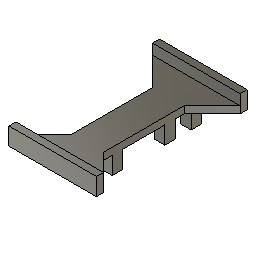
v2 (Autodesk Fusion 360 design; units mm, degrees)
Autodesk Fusion 360 part; units mm, degrees
sketch "Sketch1" plane through (0, 0, 0) normal (0, 0, 1) x (1, 0, 0) in component "Component'"
  line L0 (-12.5, 21.5) -> (12.5, 21.5)
  line L1 (12.5, 21.5) -> (12.5, 19.5)
  line L2 (12.5, 19.5) -> (-12.5, 19.5)
  line L3 (-12.5, 19.5) -> (-12.5, 21.5)
  line L4 (-12.5, -19.5) -> (12.5, -19.5)
  line L5 (12.5, -19.5) -> (12.5, -21.5)
  line L6 (12.5, -21.5) -> (-12.5, -21.5)
  line L7 (-12.5, -21.5) -> (-12.5, -19.5)
  line L8 (0, -19.5) -> (0, 19.5) construction
  line L9 (-4.5, 9) -> (-1.5, 9)
  line L10 (-1.5, 9) -> (-1.5, 6)
  line L11 (-1.5, 6) -> (-4.5, 6)
  line L12 (-4.5, 6) -> (-4.5, 9)
  line L13 (-1.5, 16.5) -> (-1.5, 13.5)
  line L14 (-1.5, 13.5) -> (-4.5, 13.5)
  line L15 (-4.5, 13.5) -> (-4.5, 16.5)
  line L16 (-4.5, 16.5) -> (-1.5, 16.5)
  line L17 (-4.5, -16.5) -> (-4.5, -13.5)
  line L18 (-1.5, -6) -> (-1.5, -9)
  line L19 (-4.5, -6) -> (-1.5, -6)
  line L20 (-4.5, -13.5) -> (-1.5, -13.5)
  line L21 (-4.5, -9) -> (-4.5, -6)
  line L22 (-1.5, -16.5) -> (-4.5, -16.5)
  line L23 (-1.5, -9) -> (-4.5, -9)
  line L24 (-1.5, -13.5) -> (-1.5, -16.5)
  line L25 (-20, 0) -> (15, 0) construction
  line L26 (4.5, 9) -> (4.5, 6)
  line L27 (4.5, 16.5) -> (4.5, 13.5)
  line L28 (1.5, 13.5) -> (1.5, 16.5)
  line L29 (4.5, -16.5) -> (1.5, -16.5)
  line L30 (4.5, -13.5) -> (4.5, -16.5)
  line L31 (1.5, -6) -> (4.5, -6)
  line L32 (4.5, -6) -> (4.5, -9)
  line L33 (1.5, -9) -> (1.5, -6)
  line L34 (1.5, -16.5) -> (1.5, -13.5)
  line L35 (1.5, 6) -> (1.5, 9)
  line L36 (1.5, 9) -> (4.5, 9)
  line L37 (4.5, 6) -> (1.5, 6)
  line L38 (4.5, -9) -> (1.5, -9)
  line L39 (1.5, 16.5) -> (4.5, 16.5)
  line L40 (1.5, -13.5) -> (4.5, -13.5)
  line L41 (4.5, 13.5) -> (1.5, 13.5)
  line L42 (4.5, 19.5) -> (4.5, -19.5)
  line L43 (-4.5, 19.5) -> (-4.5, -19.5)
  line L44 (12.5, 19.5) -> (4.5, 11.5)
  line L45 (12.5, 19.5) -> (24.453, 19.5) construction
  line L46 (-12.5, 19.5) -> (-4.5, 11.5)
  line L47 (-12.5, -19.5) -> (-4.5, -11.5)
  line L48 (12.5, -19.5) -> (4.5, -11.5)
  dimension "d1" = 39
  dimension "d2" = 25
  dimension "d3" = 2
  dimension "d6" = 3
  dimension "d7" = 3
  dimension "d8" = 1.5
  dimension "d9" = 7.5
  dimension "d10" = 3
  dimension "d11" = 3
  dimension "d12" = 7.5
  dimension "d13" = 12
  dimension "d14" = 3
  dimension "d15" = 3
  dimension "d16" = 7.5
  dimension "d17" = 3
  dimension "d18" = 3
  dimension "d19" = 7.5
  dimension "d20" = 12
  dimension "d21" = 135
  constraint horizontal L0
  constraint vertical L1
  constraint horizontal L2
  constraint vertical L3
  constraint horizontal L4
  constraint vertical L5
  constraint horizontal L6
  constraint vertical L7
  constraint equal L2 L4
  constraint equal L3 L7
  constraint coincident L4 L8.start
  constraint midpoint L2 L8.end
  constraint midpoint L4 L8.start
  constraint vertical L8
  constraint midpoint origin L8
  constraint horizontal L9
  constraint vertical L10
  constraint horizontal L11
  constraint vertical L12
  constraint horizontal L16
  constraint vertical L13
  constraint horizontal L14
  constraint vertical L15
  constraint equal L9 L16
  constraint equal L12 L15
  constraint horizontal L20
  constraint vertical L24
  constraint horizontal L22
  constraint vertical L17
  constraint horizontal L19
  constraint vertical L18
  constraint horizontal L23
  constraint vertical L21
  constraint equal L19 L20
  constraint equal L17 L21
  constraint horizontal L25
  constraint symmetric L11 L19 L25
  constraint collinear L10 L13
  constraint collinear L18 L24
  constraint collinear L10 L18
  constraint horizontal L36
  constraint vertical L26
  constraint horizontal L37
  constraint vertical L35
  constraint horizontal L39
  constraint vertical L27
  constraint horizontal L41
  constraint vertical L28
  constraint equal L36 L39
  constraint equal L28 L35
  constraint horizontal L40
  constraint vertical L30
  constraint horizontal L29
  constraint vertical L34
  constraint horizontal L31
  constraint vertical L32
  constraint horizontal L38
  constraint vertical L33
  constraint equal L31 L40
  constraint equal L33 L34
  constraint collinear L26 L27
  constraint collinear L30 L32
  constraint collinear L26 L32
  constraint symmetric L8 L10 L35
  constraint collinear L11 L37
  constraint coincident L2 L42.start
  constraint coincident L4 L42.end
  constraint perpendicular L4 L42
  constraint coincident L2 L43.start
  constraint coincident L4 L43.end
  constraint perpendicular L4 L43
  constraint collinear L26 L42
  constraint horizontal L45
  constraint coincident L42 L44.end
  constraint coincident L43 L46.end
  constraint coincident L43 L47.end
  constraint coincident L42 L48.end
  constraint symmetric L8 L44 L46
  constraint symmetric L25 L44 L48
  constraint symmetric L8 L47 L48
  measures "d1" distance of L2 L4
  measures "d2" distance of L0.start L0.end
  measures "d3" distance of L0.start L2.end
  measures "d6" distance of L13.start L15.end
  measures "d7" distance of L14.end L15.end
  measures "d8" distance of L8 L13
  measures "d9" distance of L9 L16
  measures "d10" distance of L19.start L18.start
  measures "d11" distance of L21.start L19.start
  measures "d12" distance of L19 L20
  measures "d13" distance of L11 L19
  measures "d14" distance of L28.end L27.start
  measures "d15" distance of L28.start L28.end
  measures "d16" distance of L36 L39
  measures "d17" distance of L31.start L31.end
  measures "d18" distance of L31.start L33.start
  measures "d19" distance of L31 L40
  measures "d20" distance of L31 L37
  measures "d21" angle of L44 L45
extrude "Extrude1" add sketch "Sketch1" along normal blind 2 contours L2 L15 L43 L46 | L2 L27 L42 L44 | L2 L4 L9 L10 L11 L13 L14 L16 L18 L19 L20 L22 L23 L24 L28 L29 L31 L33 L34 L35 L36 L37 L38 L39 L40 L41 L42 L43 | L13 L14 L15 L16 L43 | L9 L10 L11 L12 L43 | L27 L28 L39 L41 L42 | L26 L35 L36 L37 L42 | L18 L19 L21 L23 L43 | L31 L32 L33 L38 L42 | L4 L17 L43 L47 | L4 L30 L42 L48 | L17 L20 L22 L24 L43 | L29 L30 L34 L40 L42 in component "Component'"
extrude "Extrude2" add sketch "Sketch1" along normal blind 5 contours L0 L1 L2 L3 | L4 L5 L6 L7 in component "Component'"
extrude "Extrude3" add sketch "Sketch1" against normal blind 5 contours L13 L14 L15 L16 L43 | L9 L10 L11 L12 L43 | L27 L28 L39 L41 L42 | L26 L35 L36 L37 L42 | L18 L19 L21 L23 L43 | L31 L32 L33 L38 L42 | L17 L20 L22 L24 L43 | L29 L30 L34 L40 L42 in component "Component'"
component "Component'" placed x (1, 0, 0) y (0, 1, 0) z (0, 0, 1) at (0, 0, 0)
